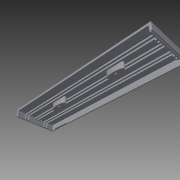
# Autodesk Inventor part: NavCom_Box_Upper_Part
Saved by Autodesk Inventor 2014 (Build 180170000, 170)
## iProperties
Created: 2019-05-25
Part Number: NavCom_Box_Upper_Part
Material: Všeobecné
Document SubType Name: Modeling
Designer: N
Density: 1 g/cm^3
Appearance: Výchozí
Author: N
Autodesk Inventor part; units mm, degrees
ref_plane "YZ Plane" through (0, 0, 0) normal (1, 0, 0) x (0, 1, 0)
ref_plane "XZ Plane" through (0, 0, 0) normal (0, 1, 0) x (-1, 0, 0)
ref_plane "XY Plane" through (0, 0, 0) normal (0, 0, 1) x (1, 0, 0)
sketch "Náčrt1" plane through (0, 0, 0) normal (0, 1, 0) x (-1, 0, 0)
  line L0 (0, 0) -> (177.8, 0)
  line L1 (177.8, 0) -> (177.8, 50.8)
  line L2 (177.8, 50.8) -> (0, 50.8)
  line L3 (0, 50.8) -> (0, 0)
  dimension "d0" = 50.8
  dimension "d1" = 177.8
  constraints: 8 end point, 2 parallel, 1 horizontal, 1 perpendicular
  measures "d0" distance between parallel lines of L0 L2
  measures "d1" distance between parallel lines of L1 L3
extrude "Vysunutí1" add sketch "Náčrt1" along normal blind 2.54
sketch "Náčrt3" plane through (0, 0, 0) normal (0, -1, 0) x (1, 0, 0)
  line L0 (0, 0) -> (-177.8, 0) projected
  line L1 (-177.8, 50.8) -> (0, 50.8) projected
  line L2 (-177.8, 50.8) -> (-175.26, 50.8)
  line L3 (-175.26, 50.8) -> (-175.26, 2.54)
  line L4 (-175.26, 2.54) -> (-2.54, 2.54)
  line L5 (-2.54, 2.54) -> (-2.54, 50.8)
  line L6 (-2.54, 50.8) -> (0, 50.8)
  line L7 (0, 50.8) -> (0, 0)
  line L8 (0, 0) -> (-177.8, 0)
  line L9 (-177.8, 0) -> (-177.8, 50.8)
  line L10 (0, 0) -> (-177.8, 0) projected
  line L11 (-177.8, 50.8) -> (-175.26, 50.8)
  dimension "d23" = 2.54
  dimension "d24" = 2.54
  dimension "d25" = 2.54
  constraints: 18 end point, 2 collinear, 1 perpendicular
  measures "d23" distance between parallel lines of L9 L3
  measures "d24" distance between parallel lines of L0 L4
  measures "d25" distance between parallel lines of L7 L5
extrude "Vysunutí2" add sketch "Náčrt3" along normal blind 6.35 contours L0 L9 L1 L3 L4 L5 L7
sketch "Náčrt4" plane through (0, -6.35, 0) normal (0, -1, 0) x (1, 0, 0)
  line L0 (0, 50.8) -> (-2.54, 50.8) projected
  line L1 (-2.54, 50.8) -> (-1.27, 50.8)
  line L2 (-1.27, 1.27) -> (-176.53, 1.27)
  line L3 (-176.53, 1.27) -> (-176.53, 50.8)
  line L4 (-176.53, 50.8) -> (-175.26, 50.8)
  line L5 (-175.26, 50.8) -> (-175.26, 2.54)
  line L6 (-175.26, 2.54) -> (-2.54, 2.54)
  line L7 (-2.54, 2.54) -> (-2.54, 50.8)
  line L8 (-1.27, 1.27) -> (-1.27, 50.8)
  line L9 (-177.8, 0) -> (0, 0) projected
  line L10 (-177.8, 50.8) -> (-177.8, 0) projected
  dimension "d26" = 1.27
  dimension "d27" = 1.27
  constraints: 16 end point, 1 midpoint
  measures "d26" distance between parallel lines of L3 L10
  measures "d27" distance between parallel lines of L9 L2
extrude "Vysunutí3" add sketch "Náčrt4" along normal blind 1.27
sketch "Náčrt5" plane through (0, 0, 0) normal (0, -1, 0) x (1, 0, 0)
  line L0 (-2.54, 2.54) -> (-2.54, 50.8) projected
  line L1 (-175.26, 50.8) -> (-2.54, 50.8) projected
  line L2 (-175.26, 50.8) -> (-175.26, 2.54) projected
  line L3 (-175.26, 41.275) -> (-2.54, 41.275)
  line L4 (-2.54, 41.275) -> (-2.54, 39.37)
  line L5 (-2.54, 39.37) -> (-175.26, 39.37)
  line L6 (-175.26, 39.37) -> (-175.26, 41.275)
  line L7 (-175.26, 2.54) -> (-175.26, 50.8) projected
  line L8 (-175.26, 37.465) -> (-2.54, 37.465)
  line L9 (-2.54, 37.465) -> (-2.54, 35.56)
  line L10 (-2.54, 35.56) -> (-175.26, 35.56)
  line L11 (-175.26, 35.56) -> (-175.26, 37.465)
  line L12 (-175.26, 28.575) -> (-2.54, 28.575)
  line L13 (-2.54, 28.575) -> (-2.54, 26.67)
  line L14 (-2.54, 26.67) -> (-175.26, 26.67)
  line L15 (-175.26, 26.67) -> (-175.26, 28.575)
  line L16 (-175.26, 24.765) -> (-2.54, 24.765)
  line L17 (-2.54, 24.765) -> (-2.54, 22.86)
  line L18 (-2.54, 22.86) -> (-175.26, 22.86)
  line L19 (-175.26, 22.86) -> (-175.26, 24.765)
  line L20 (-175.26, 15.875) -> (-2.54, 15.875)
  line L21 (-2.54, 15.875) -> (-2.54, 13.97)
  line L22 (-2.54, 13.97) -> (-175.26, 13.97)
  line L23 (-175.26, 13.97) -> (-175.26, 15.875)
  line L24 (-175.26, 12.065) -> (-2.54, 12.065)
  line L25 (-2.54, 12.065) -> (-2.54, 10.16)
  line L26 (-2.54, 10.16) -> (-175.26, 10.16)
  line L27 (-175.26, 10.16) -> (-175.26, 12.065)
  point P0 (0, 0)
  dimension "d8" = 1.905
  dimension "d10" = 1.905
  dimension "d11" = 1.905
  dimension "d12" = 1.905
  dimension "d13" = 1.905
  dimension "d14" = 1.905
  dimension "d15" = 1.905
  dimension "d16" = 1.905
  dimension "d17" = 1.905
  dimension "d18" = 11.43
  dimension "d19" = 10.795
  dimension "d20" = 10.795
  constraints: 48 end point, 12 parallel, 11 point on line, 6 horizontal, 6 perpendicular, 1 midpoint
  measures "d8" distance between parallel lines of L5 L3
  measures "d10" distance between parallel lines of L8 L10
  measures "d11" distance between parallel lines of L5 L8
  measures "d12" distance between parallel lines of L14 L12
  measures "d13" distance between parallel lines of L16 L18
  measures "d14" distance between parallel lines of L16 L14
  measures "d15" distance between parallel lines of L22 L20
  measures "d16" distance between parallel lines of L24 L26
  measures "d17" distance between parallel lines of L22 L24
  measures "d18" distance between parallel lines of L5 L1
  measures "d19" distance between parallel lines of L14 L8
  measures "d20" distance between parallel lines of L22 L16
extrude "Vysunutí4" add sketch "Náčrt5" along normal blind 1.905 contours L26 L2 L24 L0 | L22 L2 L20 L0 | L18 L2 L16 L0 | L14 L2 L12 L0 | L10 L2 L8 L0 | L5 L2 L3 L0
sketch "Náčrt6" plane through (0, -1.905, 0) normal (0, -1, 0) x (1, 0, 0)
  line L0 (-2.54, 41.275) -> (-175.26, 41.275) projected
  line L1 (-175.26, 39.37) -> (-173.3599, 39.37)
  line L2 (-173.3599, 39.37) -> (-173.3599, 41.275)
  line L3 (-173.3599, 41.275) -> (-175.26, 41.275)
  line L4 (-175.26, 41.275) -> (-175.26, 39.37)
  line L5 (-2.54, 39.37) -> (-4.4571, 39.37)
  line L6 (-4.4571, 39.37) -> (-4.4571, 41.275)
  line L7 (-4.4571, 41.275) -> (-2.54, 41.275)
  line L8 (-2.54, 41.275) -> (-2.54, 39.37)
  point P0 (0, 0)
  constraints: 16 end point, 4 parallel, 2 horizontal, 2 perpendicular, 2 point on line
extrude "Vysunutí5" add sketch "Náčrt6" along normal up to surface (5.715 mm away)
sketch "Náčrt7" plane through (0, -1.905, 0) normal (0, -1, 0) x (1, 0, 0)
  line L0 (-175.26, 35.56) -> (-175.26, 37.465) projected
  line L1 (-175.26, 35.56) -> (-2.54, 35.56) projected
  line L2 (-2.54, 37.465) -> (-175.26, 37.465) projected
  line L3 (-175.26, 37.465) -> (-173.3424, 37.465)
  line L4 (-173.3424, 37.465) -> (-173.3424, 35.56)
  line L5 (-173.3424, 35.56) -> (-175.26, 35.56)
  line L6 (-175.26, 35.56) -> (-175.26, 37.465)
  line L7 (-2.54, 35.56) -> (-4.4396, 35.56)
  line L8 (-4.4396, 35.56) -> (-4.4396, 37.465)
  line L9 (-4.4396, 37.465) -> (-2.54, 37.465)
  line L10 (-2.54, 37.465) -> (-2.54, 35.56)
  point P0 (0, 0)
  constraints: 16 end point, 4 parallel, 2 horizontal, 2 perpendicular, 2 point on line
extrude "Vysunutí6" add sketch "Náčrt7" along normal up to surface (5.715 mm away) contours L0 L2 L4 L1 | L8 L2 L10 L1
sketch "Náčrt10" plane through (0, -1.905, 0) normal (0, -1, 0) x (1, 0, 0)
  line L0 (-2.54, 13.97) -> (-175.26, 13.97) projected
  line L1 (-175.26, 15.875) -> (-173.3527, 15.875)
  line L2 (-173.3527, 15.875) -> (-173.3527, 13.97)
  line L3 (-173.3527, 13.97) -> (-175.26, 13.97)
  line L4 (-175.26, 13.97) -> (-175.26, 15.875)
  line L5 (-2.54, 15.875) -> (-4.4457, 15.875)
  line L6 (-4.4457, 15.875) -> (-4.4457, 13.97)
  line L7 (-4.4457, 13.97) -> (-2.54, 13.97)
  line L8 (-2.54, 13.97) -> (-2.54, 15.875)
  point P0 (0, 0)
  constraints: 16 end point, 4 parallel, 2 horizontal, 2 perpendicular, 2 point on line
extrude "Vysunutí9" add sketch "Náčrt10" along normal up to surface (5.715 mm away)
sketch "Náčrt11" plane through (0, -1.905, 0) normal (0, -1, 0) x (1, 0, 0)
  line L0 (-175.26, 10.16) -> (-2.54, 10.16) projected
  line L1 (-175.26, 12.065) -> (-173.3599, 12.065)
  line L2 (-173.3599, 12.065) -> (-173.3599, 10.16)
  line L3 (-173.3599, 10.16) -> (-175.26, 10.16)
  line L4 (-175.26, 10.16) -> (-175.26, 12.065)
  line L5 (-2.54, 12.065) -> (-4.4431, 12.065)
  line L6 (-4.4431, 12.065) -> (-4.4431, 10.16)
  line L7 (-4.4431, 10.16) -> (-2.54, 10.16)
  line L8 (-2.54, 10.16) -> (-2.54, 12.065)
  point P0 (0, 0)
  constraints: 16 end point, 4 parallel, 2 horizontal, 2 perpendicular, 2 point on line
extrude "Vysunutí10" add sketch "Náčrt11" along normal up to surface (5.715 mm away)
sketch "Náčrt12" plane through (0, 0, 0) normal (0, -1, 0) x (1, 0, 0)
  line L0 (-2.54, 35.56) -> (-175.26, 35.56) projected
  line L1 (-175.26, 35.56) -> (-175.26, 28.575) projected
  ellipse E0 centre (-127, 32.0675) end of major axis (-116.84, 32.0675) minor radius 3.175
  line L2 (-175.26, 50.8) -> (-2.54, 50.8) projected
  ellipse E1 centre (-50.8, 32.0675) end of major axis (-40.64, 32.0675) minor radius 3.175
  point P0 (0, 0)
  dimension "d42" = 10.16
  dimension "d43" = 3.175
  dimension "d45" = 10.16
  dimension "d46" = 3.175
  dimension "d40" = 48.26
  dimension "d41" = 18.7325
  dimension "d44" = 76.2
  dimension "d47" = 0
  constraints: 2 horizontal, 4 other
  measures "d40" distance from line of L1 point (-127, 32.068)
  measures "d41" distance from line of point (-127, 32.068) L2
  measures "d44" distance of point (-50.8, 32.068) point (-127, 32.068)
  measures "d47" vertical distance of point (-50.8, 32.068) point (-127, 32.068)
extrude "Vysunutí11" add sketch "Náčrt12" along normal up to surface (7.62 mm away)
sketch "Náčrt13" plane through (-127, -7.62, 32.0675) normal (0, -1, 0) x (1, 0, 0)
  ellipse E0 centre (0, 0) end of major axis (-10.16, 0) minor radius 3.175 projected
  circle A0 centre (0, 0) radius 0.9525
  point P0 (127, -32.0675)
  dimension "d50" = 1.905
  constraints: 1 centre point, 1 coincident, 1 other
  measures "d50" diameter of A0
extrude "Vysunutí12" cut sketch "Náčrt13" against normal through all contours A0
sketch "Náčrt14" plane through (-50.8, -7.62, 32.0675) normal (0, -1, 0) x (1, 0, 0)
  ellipse E0 centre (0, 0) end of major axis (-10.16, 0) minor radius 3.175 projected
  circle A0 centre (0, 0) radius 0.9525
  point P0 (50.8, -32.0675)
  dimension "d53" = 1.905
  constraints: 1 centre point, 1 coincident, 1 other
  measures "d53" diameter of A0
extrude "Vysunutí13" cut sketch "Náčrt14" against normal through all contours A0
sketch "Náčrt15" plane through (0, 2.54, 0) normal (0, 1, 0) x (1, 0, 0)
  circle A0 centre (-50.8, -32.0675) radius 0.9525 projected
  circle A1 centre (-127, -32.0675) radius 0.9525 projected
  circle A2 centre (-127, -32.0675) radius 2.667
  circle A3 centre (-50.8, -32.0675) radius 2.667
  dimension "d56" = 5.334
  dimension "d57" = 5.334
  constraints: 2 centre point, 2 coincident
  measures "d56" diameter of A2
  measures "d57" diameter of A3
extrude "Vysunutí14" cut sketch "Náčrt15" against normal blind 2.54
sketch "Náčrt16" plane through (0, -7.62, 0) normal (0, -1, 0) x (1, 0, 0)
  line L0 (-2.54, 2.54) -> (-175.26, 2.54) projected
  line L1 (-175.26, 2.54) -> (-175.26, 10.16) projected
  line L2 (-176.53, 1.27) -> (-1.27, 1.27) projected
  line L3 (-170.18, 2.54) -> (-149.86, 2.54)
  line L4 (-149.86, 2.54) -> (-149.86, 1.27)
  line L5 (-149.86, 1.27) -> (-170.18, 1.27)
  line L6 (-170.18, 1.27) -> (-170.18, 2.54)
  point P0 (0, 0)
  dimension "d60" = 20.32
  dimension "d61" = 25.4
  constraints: 8 end point, 2 parallel, 2 point on line, 1 horizontal, 1 perpendicular
  measures "d60" distance between parallel lines of L4 L6
  measures "d61" distance between parallel lines of L4 L1
extrude "Vysunutí15" cut sketch "Náčrt16" against normal up to surface (1.27 mm away)
